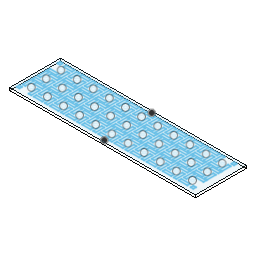
Cable Housing v2 (Autodesk Fusion 360 archive; units mm, degrees)
design "shelf small"
Autodesk Fusion 360 part; units mm, degrees
sketch "Sketch1" plane through (0, 0, 0) normal (0, 0, 1) x (1, 0, 0)
  line L0 (109.5, -30) -> (-109.5, -30)
  line L1 (-109.5, -30) -> (-109.5, 30)
  line L2 (-109.5, 30) -> (109.5, 30)
  line L3 (109.5, 30) -> (109.5, -30)
  line L4 (109.5, -30) -> (-109.5, 30) construction
  line L5 (-109.5, -30) -> (109.5, 30) construction
  dimension "d1" = 60
  dimension "d2" = 219
  constraint horizontal L0
  constraint perpendicular L0 L1
  constraint parallel L0 L2
  constraint parallel L1 L3
  constraint coincident L4 origin
  constraint coincident L5 origin
  measures "d1" distance of L0.end L1.end
  measures "d2" distance of L1.end L2.end
extrude "Extrude1" add sketch "Sketch1" along normal blind 3
sketch "Sketch5" plane through (0, 0, 3) normal (0, 0, 1) x (-1, 0, 0)
  line L0 (-109.5, -30) -> (109.5, -30)
  line L1 (109.5, -30) -> (109.5, 30)
  line L2 (109.5, 30) -> (-109.5, 30)
  line L3 (-109.5, 30) -> (-109.5, -30)
  circle A0 centre (97, 17) radius 1.5
  line L4 (99, 9) -> (89, 9)
  line L5 (89, 9) -> (89, 12)
  line L6 (89, 12) -> (99, 12)
  line L7 (99, 12) -> (99, 9)
  line L8 (92, 15) -> (89, 15)
  line L9 (89, 15) -> (89, 25)
  line L10 (89, 25) -> (92, 25)
  line L11 (92, 25) -> (92, 15)
  line L12 (102, 19) -> (105, 19)
  line L13 (105, 19) -> (105, 9)
  line L14 (105, 9) -> (102, 9)
  line L15 (102, 9) -> (102, 19)
  line L16 (70, 15) -> (70, 25)
  line L17 (73, 25) -> (73, 15)
  line L18 (73, 15) -> (70, 15)
  line L19 (70, 9) -> (70, 12)
  line L20 (86, 9) -> (83, 9)
  line L21 (83, 9) -> (83, 19)
  line L22 (86, 19) -> (86, 9)
  line L23 (83, 19) -> (86, 19)
  line L24 (76, 25) -> (76, 22)
  line L25 (86, 25) -> (76, 25)
  line L26 (86, 22) -> (86, 25)
  line L27 (70, 12) -> (80, 12)
  line L28 (80, 9) -> (70, 9)
  line L29 (80, 12) -> (80, 9)
  circle A1 centre (78, 17) radius 1.5
  line L30 (76, 22) -> (86, 22)
  line L31 (70, 25) -> (73, 25)
  line L32 (51, 15) -> (51, 25)
  line L33 (54, 25) -> (54, 15)
  line L34 (54, 15) -> (51, 15)
  line L35 (51, 9) -> (51, 12)
  line L36 (67, 9) -> (64, 9)
  line L37 (64, 9) -> (64, 19)
  line L38 (67, 19) -> (67, 9)
  line L39 (64, 19) -> (67, 19)
  line L40 (57, 25) -> (57, 22)
  line L41 (67, 25) -> (57, 25)
  line L42 (67, 22) -> (67, 25)
  line L43 (51, 12) -> (61, 12)
  line L44 (61, 9) -> (51, 9)
  line L45 (61, 12) -> (61, 9)
  circle A2 centre (59, 17) radius 1.5
  line L46 (57, 22) -> (67, 22)
  line L47 (51, 25) -> (54, 25)
  line L48 (32, 15) -> (32, 25)
  line L49 (35, 25) -> (35, 15)
  line L50 (35, 15) -> (32, 15)
  line L51 (32, 9) -> (32, 12)
  line L52 (48, 9) -> (45, 9)
  line L53 (45, 9) -> (45, 19)
  line L54 (48, 19) -> (48, 9)
  line L55 (45, 19) -> (48, 19)
  line L56 (38, 25) -> (38, 22)
  line L57 (48, 25) -> (38, 25)
  line L58 (48, 22) -> (48, 25)
  line L59 (32, 12) -> (42, 12)
  line L60 (42, 9) -> (32, 9)
  line L61 (42, 12) -> (42, 9)
  circle A3 centre (40, 17) radius 1.5
  line L62 (38, 22) -> (48, 22)
  line L63 (32, 25) -> (35, 25)
  line L64 (13, 15) -> (13, 25)
  line L65 (16, 25) -> (16, 15)
  line L66 (16, 15) -> (13, 15)
  line L67 (13, 9) -> (13, 12)
  line L68 (29, 9) -> (26, 9)
  line L69 (26, 9) -> (26, 19)
  line L70 (29, 19) -> (29, 9)
  line L71 (26, 19) -> (29, 19)
  line L72 (19, 25) -> (19, 22)
  line L73 (29, 25) -> (19, 25)
  line L74 (29, 22) -> (29, 25)
  line L75 (13, 12) -> (23, 12)
  line L76 (23, 9) -> (13, 9)
  line L77 (23, 12) -> (23, 9)
  circle A4 centre (21, 17) radius 1.5
  line L78 (19, 22) -> (29, 22)
  line L79 (13, 25) -> (16, 25)
  line L80 (-6, 15) -> (-6, 25)
  line L81 (-3, 25) -> (-3, 15)
  line L82 (-3, 15) -> (-6, 15)
  line L83 (-6, 9) -> (-6, 12)
  line L84 (10, 9) -> (7, 9)
  line L85 (7, 9) -> (7, 19)
  line L86 (10, 19) -> (10, 9)
  line L87 (7, 19) -> (10, 19)
  line L88 (0, 25) -> (0, 22)
  line L89 (10, 25) -> (0, 25)
  line L90 (10, 22) -> (10, 25)
  line L91 (-6, 12) -> (4, 12)
  line L92 (4, 9) -> (-6, 9)
  line L93 (4, 12) -> (4, 9)
  circle A5 centre (2, 17) radius 1.5
  line L94 (0, 22) -> (10, 22)
  line L95 (-6, 25) -> (-3, 25)
  line L96 (-25, 15) -> (-25, 25)
  line L97 (-22, 25) -> (-22, 15)
  line L98 (-22, 15) -> (-25, 15)
  line L99 (-25, 9) -> (-25, 12)
  line L100 (-9, 9) -> (-12, 9)
  line L101 (-12, 9) -> (-12, 19)
  line L102 (-9, 19) -> (-9, 9)
  line L103 (-12, 19) -> (-9, 19)
  line L104 (-19, 25) -> (-19, 22)
  line L105 (-9, 25) -> (-19, 25)
  line L106 (-9, 22) -> (-9, 25)
  line L107 (-25, 12) -> (-15, 12)
  line L108 (-15, 9) -> (-25, 9)
  line L109 (-15, 12) -> (-15, 9)
  circle A6 centre (-17, 17) radius 1.5
  line L110 (-19, 22) -> (-9, 22)
  line L111 (-25, 25) -> (-22, 25)
  line L112 (-44, 15) -> (-44, 25)
  line L113 (-41, 25) -> (-41, 15)
  line L114 (-41, 15) -> (-44, 15)
  line L115 (-44, 9) -> (-44, 12)
  line L116 (-28, 9) -> (-31, 9)
  line L117 (-31, 9) -> (-31, 19)
  line L118 (-28, 19) -> (-28, 9)
  line L119 (-31, 19) -> (-28, 19)
  line L120 (-38, 25) -> (-38, 22)
  line L121 (-28, 25) -> (-38, 25)
  line L122 (-28, 22) -> (-28, 25)
  line L123 (-44, 12) -> (-34, 12)
  line L124 (-34, 9) -> (-44, 9)
  line L125 (-34, 12) -> (-34, 9)
  circle A7 centre (-36, 17) radius 1.5
  line L126 (-38, 22) -> (-28, 22)
  line L127 (-44, 25) -> (-41, 25)
  line L128 (-63, 15) -> (-63, 25)
  line L129 (-60, 25) -> (-60, 15)
  line L130 (-60, 15) -> (-63, 15)
  line L131 (-63, 9) -> (-63, 12)
  line L132 (-47, 9) -> (-50, 9)
  line L133 (-50, 9) -> (-50, 19)
  line L134 (-47, 19) -> (-47, 9)
  line L135 (-50, 19) -> (-47, 19)
  line L136 (-57, 25) -> (-57, 22)
  line L137 (-47, 25) -> (-57, 25)
  line L138 (-47, 22) -> (-47, 25)
  line L139 (-63, 12) -> (-53, 12)
  line L140 (-53, 9) -> (-63, 9)
  line L141 (-53, 12) -> (-53, 9)
  circle A8 centre (-55, 17) radius 1.5
  line L142 (-57, 22) -> (-47, 22)
  line L143 (-63, 25) -> (-60, 25)
  line L144 (-82, 15) -> (-82, 25)
  line L145 (-79, 25) -> (-79, 15)
  line L146 (-79, 15) -> (-82, 15)
  line L147 (-82, 9) -> (-82, 12)
  line L148 (-66, 9) -> (-69, 9)
  line L149 (-69, 9) -> (-69, 19)
  line L150 (-66, 19) -> (-66, 9)
  line L151 (-69, 19) -> (-66, 19)
  line L152 (-76, 25) -> (-76, 22)
  line L153 (-66, 25) -> (-76, 25)
  line L154 (-66, 22) -> (-66, 25)
  line L155 (-82, 12) -> (-72, 12)
  line L156 (-72, 9) -> (-82, 9)
  line L157 (-72, 12) -> (-72, 9)
  circle A9 centre (-74, 17) radius 1.5
  line L158 (-76, 22) -> (-66, 22)
  line L159 (-82, 25) -> (-79, 25)
  line L160 (-101, 9) -> (-101, 12)
  line L161 (-85, 9) -> (-88, 9)
  line L162 (-88, 9) -> (-88, 19)
  line L163 (-85, 19) -> (-85, 9)
  line L164 (-88, 19) -> (-85, 19)
  line L165 (-95, 25) -> (-95, 22)
  line L166 (-85, 25) -> (-95, 25)
  line L167 (-85, 22) -> (-85, 25)
  line L168 (-101, 12) -> (-91, 12)
  line L169 (-91, 9) -> (-101, 9)
  line L170 (-91, 12) -> (-91, 9)
  circle A10 centre (-93, 17) radius 1.5
  line L171 (-95, 22) -> (-85, 22)
  line L172 (89, -2.5) -> (89, 7.5)
  line L173 (92, 7.5) -> (92, -2.5)
  line L174 (92, -2.5) -> (89, -2.5)
  line L175 (89, -8.5) -> (89, -5.5)
  line L176 (105, -8.5) -> (102, -8.5)
  line L177 (102, -8.5) -> (102, 1.5)
  line L178 (105, 1.5) -> (105, -8.5)
  line L179 (102, 1.5) -> (105, 1.5)
  line L180 (95, 7.5) -> (95, 4.5)
  line L181 (105, 7.5) -> (95, 7.5)
  line L182 (105, 4.5) -> (105, 7.5)
  line L183 (89, -5.5) -> (99, -5.5)
  line L184 (99, -8.5) -> (89, -8.5)
  line L185 (99, -5.5) -> (99, -8.5)
  circle A11 centre (97, -0.5) radius 1.5
  line L186 (95, 4.5) -> (105, 4.5)
  line L187 (89, 7.5) -> (92, 7.5)
  line L188 (70, -2.5) -> (70, 7.5)
  line L189 (73, 7.5) -> (73, -2.5)
  line L190 (73, -2.5) -> (70, -2.5)
  line L191 (70, -8.5) -> (70, -5.5)
  line L192 (86, -8.5) -> (83, -8.5)
  line L193 (83, -8.5) -> (83, 1.5)
  line L194 (86, 1.5) -> (86, -8.5)
  line L195 (83, 1.5) -> (86, 1.5)
  line L196 (76, 7.5) -> (76, 4.5)
  line L197 (86, 7.5) -> (76, 7.5)
  line L198 (86, 4.5) -> (86, 7.5)
  line L199 (70, -5.5) -> (80, -5.5)
  line L200 (80, -8.5) -> (70, -8.5)
  line L201 (80, -5.5) -> (80, -8.5)
  circle A12 centre (78, -0.5) radius 1.5
  line L202 (76, 4.5) -> (86, 4.5)
  line L203 (70, 7.5) -> (73, 7.5)
  line L204 (51, -2.5) -> (51, 7.5)
  line L205 (54, 7.5) -> (54, -2.5)
  line L206 (54, -2.5) -> (51, -2.5)
  line L207 (51, -8.5) -> (51, -5.5)
  line L208 (67, -8.5) -> (64, -8.5)
  line L209 (64, -8.5) -> (64, 1.5)
  line L210 (67, 1.5) -> (67, -8.5)
  line L211 (64, 1.5) -> (67, 1.5)
  line L212 (57, 7.5) -> (57, 4.5)
  line L213 (67, 7.5) -> (57, 7.5)
  line L214 (67, 4.5) -> (67, 7.5)
  line L215 (51, -5.5) -> (61, -5.5)
  line L216 (61, -8.5) -> (51, -8.5)
  line L217 (61, -5.5) -> (61, -8.5)
  circle A13 centre (59, -0.5) radius 1.5
  line L218 (57, 4.5) -> (67, 4.5)
  line L219 (51, 7.5) -> (54, 7.5)
  line L220 (32, -2.5) -> (32, 7.5)
  line L221 (35, 7.5) -> (35, -2.5)
  line L222 (35, -2.5) -> (32, -2.5)
  line L223 (32, -8.5) -> (32, -5.5)
  line L224 (48, -8.5) -> (45, -8.5)
  line L225 (45, -8.5) -> (45, 1.5)
  line L226 (48, 1.5) -> (48, -8.5)
  line L227 (45, 1.5) -> (48, 1.5)
  line L228 (38, 7.5) -> (38, 4.5)
  line L229 (48, 7.5) -> (38, 7.5)
  line L230 (48, 4.5) -> (48, 7.5)
  line L231 (32, -5.5) -> (42, -5.5)
  line L232 (42, -8.5) -> (32, -8.5)
  line L233 (42, -5.5) -> (42, -8.5)
  circle A14 centre (40, -0.5) radius 1.5
  line L234 (38, 4.5) -> (48, 4.5)
  line L235 (32, 7.5) -> (35, 7.5)
  line L236 (13, -2.5) -> (13, 7.5)
  line L237 (16, 7.5) -> (16, -2.5)
  line L238 (16, -2.5) -> (13, -2.5)
  line L239 (13, -8.5) -> (13, -5.5)
  line L240 (29, -8.5) -> (26, -8.5)
  line L241 (26, -8.5) -> (26, 1.5)
  line L242 (29, 1.5) -> (29, -8.5)
  line L243 (26, 1.5) -> (29, 1.5)
  line L244 (19, 7.5) -> (19, 4.5)
  line L245 (29, 7.5) -> (19, 7.5)
  line L246 (29, 4.5) -> (29, 7.5)
  line L247 (13, -5.5) -> (23, -5.5)
  line L248 (23, -8.5) -> (13, -8.5)
  line L249 (23, -5.5) -> (23, -8.5)
  circle A15 centre (21, -0.5) radius 1.5
  line L250 (19, 4.5) -> (29, 4.5)
  line L251 (13, 7.5) -> (16, 7.5)
  line L252 (-6, -2.5) -> (-6, 7.5)
  line L253 (-3, 7.5) -> (-3, -2.5)
  line L254 (-3, -2.5) -> (-6, -2.5)
  line L255 (-6, -8.5) -> (-6, -5.5)
  line L256 (10, -8.5) -> (7, -8.5)
  line L257 (7, -8.5) -> (7, 1.5)
  line L258 (10, 1.5) -> (10, -8.5)
  line L259 (7, 1.5) -> (10, 1.5)
  line L260 (0, 7.5) -> (0, 4.5)
  line L261 (10, 7.5) -> (0, 7.5)
  line L262 (10, 4.5) -> (10, 7.5)
  line L263 (-6, -5.5) -> (4, -5.5)
  line L264 (4, -8.5) -> (-6, -8.5)
  line L265 (4, -5.5) -> (4, -8.5)
  circle A16 centre (2, -0.5) radius 1.5
  line L266 (0, 4.5) -> (10, 4.5)
  line L267 (-6, 7.5) -> (-3, 7.5)
  line L268 (-25, -2.5) -> (-25, 7.5)
  line L269 (-22, 7.5) -> (-22, -2.5)
  line L270 (-22, -2.5) -> (-25, -2.5)
  line L271 (-25, -8.5) -> (-25, -5.5)
  line L272 (-9, -8.5) -> (-12, -8.5)
  line L273 (-12, -8.5) -> (-12, 1.5)
  line L274 (-9, 1.5) -> (-9, -8.5)
  line L275 (-12, 1.5) -> (-9, 1.5)
  line L276 (-19, 7.5) -> (-19, 4.5)
  line L277 (-9, 7.5) -> (-19, 7.5)
  line L278 (-9, 4.5) -> (-9, 7.5)
  line L279 (-25, -5.5) -> (-15, -5.5)
  line L280 (-15, -8.5) -> (-25, -8.5)
  line L281 (-15, -5.5) -> (-15, -8.5)
  circle A17 centre (-17, -0.5) radius 1.5
  line L282 (-19, 4.5) -> (-9, 4.5)
  line L283 (-25, 7.5) -> (-22, 7.5)
  line L284 (-44, -2.5) -> (-44, 7.5)
  line L285 (-41, 7.5) -> (-41, -2.5)
  line L286 (-41, -2.5) -> (-44, -2.5)
  line L287 (-44, -8.5) -> (-44, -5.5)
  line L288 (-28, -8.5) -> (-31, -8.5)
  line L289 (-31, -8.5) -> (-31, 1.5)
  line L290 (-28, 1.5) -> (-28, -8.5)
  line L291 (-31, 1.5) -> (-28, 1.5)
  line L292 (-38, 7.5) -> (-38, 4.5)
  line L293 (-28, 7.5) -> (-38, 7.5)
  line L294 (-28, 4.5) -> (-28, 7.5)
  line L295 (-44, -5.5) -> (-34, -5.5)
  line L296 (-34, -8.5) -> (-44, -8.5)
  line L297 (-34, -5.5) -> (-34, -8.5)
  circle A18 centre (-36, -0.5) radius 1.5
  line L298 (-38, 4.5) -> (-28, 4.5)
  line L299 (-44, 7.5) -> (-41, 7.5)
  line L300 (-63, -2.5) -> (-63, 7.5)
  line L301 (-60, 7.5) -> (-60, -2.5)
  line L302 (-60, -2.5) -> (-63, -2.5)
  line L303 (-63, -8.5) -> (-63, -5.5)
  line L304 (-47, -8.5) -> (-50, -8.5)
  line L305 (-50, -8.5) -> (-50, 1.5)
  line L306 (-47, 1.5) -> (-47, -8.5)
  line L307 (-50, 1.5) -> (-47, 1.5)
  line L308 (-57, 7.5) -> (-57, 4.5)
  line L309 (-47, 7.5) -> (-57, 7.5)
  line L310 (-47, 4.5) -> (-47, 7.5)
  line L311 (-63, -5.5) -> (-53, -5.5)
  line L312 (-53, -8.5) -> (-63, -8.5)
  line L313 (-53, -5.5) -> (-53, -8.5)
  circle A19 centre (-55, -0.5) radius 1.5
  line L314 (-57, 4.5) -> (-47, 4.5)
  line L315 (-63, 7.5) -> (-60, 7.5)
  line L316 (-82, -2.5) -> (-82, 7.5)
  line L317 (-79, 7.5) -> (-79, -2.5)
  line L318 (-79, -2.5) -> (-82, -2.5)
  line L319 (-82, -8.5) -> (-82, -5.5)
  line L320 (-66, -8.5) -> (-69, -8.5)
  line L321 (-69, -8.5) -> (-69, 1.5)
  line L322 (-66, 1.5) -> (-66, -8.5)
  line L323 (-69, 1.5) -> (-66, 1.5)
  line L324 (-76, 7.5) -> (-76, 4.5)
  line L325 (-66, 7.5) -> (-76, 7.5)
  line L326 (-66, 4.5) -> (-66, 7.5)
  line L327 (-82, -5.5) -> (-72, -5.5)
  line L328 (-72, -8.5) -> (-82, -8.5)
  line L329 (-72, -5.5) -> (-72, -8.5)
  circle A20 centre (-74, -0.5) radius 1.5
  line L330 (-76, 4.5) -> (-66, 4.5)
  line L331 (-82, 7.5) -> (-79, 7.5)
  line L332 (-101, -2.5) -> (-101, 7.5)
  line L333 (-98, 7.5) -> (-98, -2.5)
  line L334 (-98, -2.5) -> (-101, -2.5)
  line L335 (-101, -8.5) -> (-101, -5.5)
  line L336 (-85, -8.5) -> (-88, -8.5)
  line L337 (-88, -8.5) -> (-88, 1.5)
  line L338 (-85, 1.5) -> (-85, -8.5)
  line L339 (-88, 1.5) -> (-85, 1.5)
  line L340 (-95, 7.5) -> (-95, 4.5)
  line L341 (-85, 7.5) -> (-95, 7.5)
  line L342 (-85, 4.5) -> (-85, 7.5)
  line L343 (-101, -5.5) -> (-91, -5.5)
  line L344 (-91, -8.5) -> (-101, -8.5)
  line L345 (-91, -5.5) -> (-91, -8.5)
  circle A21 centre (-93, -0.5) radius 1.5
  line L346 (-95, 4.5) -> (-85, 4.5)
  line L347 (-101, 7.5) -> (-98, 7.5)
  line L348 (89, -20) -> (89, -10)
  line L349 (92, -10) -> (92, -20)
  line L350 (92, -20) -> (89, -20)
  line L351 (89, -26) -> (89, -23)
  line L352 (95, -10) -> (95, -13)
  line L353 (105, -10) -> (95, -10)
  line L354 (105, -13) -> (105, -10)
  line L355 (89, -23) -> (99, -23)
  line L356 (99, -26) -> (89, -26)
  line L357 (99, -23) -> (99, -26)
  circle A22 centre (97, -18) radius 1.5
  line L358 (95, -13) -> (105, -13)
  line L359 (89, -10) -> (92, -10)
  line L360 (70, -20) -> (70, -10)
  line L361 (73, -10) -> (73, -20)
  line L362 (73, -20) -> (70, -20)
  line L363 (70, -26) -> (70, -23)
  line L364 (86, -26) -> (83, -26)
  line L365 (83, -26) -> (83, -16)
  line L366 (86, -16) -> (86, -26)
  line L367 (83, -16) -> (86, -16)
  line L368 (76, -10) -> (76, -13)
  line L369 (86, -10) -> (76, -10)
  line L370 (86, -13) -> (86, -10)
  line L371 (70, -23) -> (80, -23)
  line L372 (80, -26) -> (70, -26)
  line L373 (80, -23) -> (80, -26)
  circle A23 centre (78, -18) radius 1.5
  line L374 (76, -13) -> (86, -13)
  line L375 (70, -10) -> (73, -10)
  line L376 (51, -20) -> (51, -10)
  line L377 (54, -10) -> (54, -20)
  line L378 (54, -20) -> (51, -20)
  line L379 (51, -26) -> (51, -23)
  line L380 (67, -26) -> (64, -26)
  line L381 (64, -26) -> (64, -16)
  line L382 (67, -16) -> (67, -26)
  line L383 (64, -16) -> (67, -16)
  line L384 (57, -10) -> (57, -13)
  line L385 (67, -10) -> (57, -10)
  line L386 (67, -13) -> (67, -10)
  line L387 (51, -23) -> (61, -23)
  line L388 (61, -26) -> (51, -26)
  line L389 (61, -23) -> (61, -26)
  circle A24 centre (59, -18) radius 1.5
  line L390 (57, -13) -> (67, -13)
  line L391 (51, -10) -> (54, -10)
  line L392 (32, -20) -> (32, -10)
  line L393 (35, -10) -> (35, -20)
  line L394 (35, -20) -> (32, -20)
  line L395 (32, -26) -> (32, -23)
  line L396 (48, -26) -> (45, -26)
  line L397 (45, -26) -> (45, -16)
  line L398 (48, -16) -> (48, -26)
  line L399 (45, -16) -> (48, -16)
  line L400 (38, -10) -> (38, -13)
  line L401 (48, -10) -> (38, -10)
  line L402 (48, -13) -> (48, -10)
  line L403 (32, -23) -> (42, -23)
  line L404 (42, -26) -> (32, -26)
  line L405 (42, -23) -> (42, -26)
  circle A25 centre (40, -18) radius 1.5
  line L406 (38, -13) -> (48, -13)
  line L407 (32, -10) -> (35, -10)
  line L408 (13, -20) -> (13, -10)
  line L409 (16, -10) -> (16, -20)
  line L410 (16, -20) -> (13, -20)
  line L411 (13, -26) -> (13, -23)
  line L412 (29, -26) -> (26, -26)
  line L413 (26, -26) -> (26, -16)
  line L414 (29, -16) -> (29, -26)
  line L415 (26, -16) -> (29, -16)
  line L416 (19, -10) -> (19, -13)
  line L417 (29, -10) -> (19, -10)
  line L418 (29, -13) -> (29, -10)
  line L419 (13, -23) -> (23, -23)
  line L420 (23, -26) -> (13, -26)
  line L421 (23, -23) -> (23, -26)
  circle A26 centre (21, -18) radius 1.5
  line L422 (19, -13) -> (29, -13)
  line L423 (13, -10) -> (16, -10)
  line L424 (-6, -20) -> (-6, -10)
  line L425 (-3, -10) -> (-3, -20)
  line L426 (-3, -20) -> (-6, -20)
  line L427 (-6, -26) -> (-6, -23)
  line L428 (10, -26) -> (7, -26)
  line L429 (7, -26) -> (7, -16)
  line L430 (10, -16) -> (10, -26)
  line L431 (7, -16) -> (10, -16)
  line L432 (0, -10) -> (0, -13)
  line L433 (10, -10) -> (0, -10)
  line L434 (10, -13) -> (10, -10)
  line L435 (-6, -23) -> (4, -23)
  line L436 (4, -26) -> (-6, -26)
  line L437 (4, -23) -> (4, -26)
  circle A27 centre (2, -18) radius 1.5
  line L438 (0, -13) -> (10, -13)
  line L439 (-6, -10) -> (-3, -10)
  line L440 (-25, -20) -> (-25, -10)
  line L441 (-22, -10) -> (-22, -20)
  line L442 (-22, -20) -> (-25, -20)
  line L443 (-25, -26) -> (-25, -23)
  line L444 (-9, -26) -> (-12, -26)
  line L445 (-12, -26) -> (-12, -16)
  line L446 (-9, -16) -> (-9, -26)
  line L447 (-12, -16) -> (-9, -16)
  line L448 (-19, -10) -> (-19, -13)
  line L449 (-9, -10) -> (-19, -10)
  line L450 (-9, -13) -> (-9, -10)
  line L451 (-25, -23) -> (-15, -23)
  line L452 (-15, -26) -> (-25, -26)
  line L453 (-15, -23) -> (-15, -26)
  circle A28 centre (-17, -18) radius 1.5
  line L454 (-19, -13) -> (-9, -13)
  line L455 (-25, -10) -> (-22, -10)
  line L456 (-44, -20) -> (-44, -10)
  line L457 (-41, -10) -> (-41, -20)
  line L458 (-41, -20) -> (-44, -20)
  line L459 (-44, -26) -> (-44, -23)
  line L460 (-28, -26) -> (-31, -26)
  line L461 (-31, -26) -> (-31, -16)
  line L462 (-28, -16) -> (-28, -26)
  line L463 (-31, -16) -> (-28, -16)
  line L464 (-38, -10) -> (-38, -13)
  line L465 (-28, -10) -> (-38, -10)
  line L466 (-28, -13) -> (-28, -10)
  line L467 (-44, -23) -> (-34, -23)
  line L468 (-34, -26) -> (-44, -26)
  line L469 (-34, -23) -> (-34, -26)
  circle A29 centre (-36, -18) radius 1.5
  line L470 (-38, -13) -> (-28, -13)
  line L471 (-44, -10) -> (-41, -10)
  line L472 (-63, -20) -> (-63, -10)
  line L473 (-60, -10) -> (-60, -20)
  line L474 (-60, -20) -> (-63, -20)
  line L475 (-63, -26) -> (-63, -23)
  line L476 (-47, -26) -> (-50, -26)
  line L477 (-50, -26) -> (-50, -16)
  line L478 (-47, -16) -> (-47, -26)
  line L479 (-50, -16) -> (-47, -16)
  line L480 (-57, -10) -> (-57, -13)
  line L481 (-47, -10) -> (-57, -10)
  line L482 (-47, -13) -> (-47, -10)
  line L483 (-63, -23) -> (-53, -23)
  line L484 (-53, -26) -> (-63, -26)
  line L485 (-53, -23) -> (-53, -26)
  circle A30 centre (-55, -18) radius 1.5
  line L486 (-57, -13) -> (-47, -13)
  line L487 (-63, -10) -> (-60, -10)
  line L488 (-82, -20) -> (-82, -10)
  line L489 (-79, -10) -> (-79, -20)
  line L490 (-79, -20) -> (-82, -20)
  line L491 (-82, -26) -> (-82, -23)
  line L492 (-66, -26) -> (-69, -26)
  line L493 (-69, -26) -> (-69, -16)
  line L494 (-66, -16) -> (-66, -26)
  line L495 (-69, -16) -> (-66, -16)
  line L496 (-76, -10) -> (-76, -13)
  line L497 (-66, -10) -> (-76, -10)
  line L498 (-66, -13) -> (-66, -10)
  line L499 (-82, -23) -> (-72, -23)
  line L500 (-72, -26) -> (-82, -26)
  line L501 (-72, -23) -> (-72, -26)
  circle A31 centre (-74, -18) radius 1.5
  line L502 (-76, -13) -> (-66, -13)
  line L503 (-82, -10) -> (-79, -10)
  line L504 (-101, -20) -> (-101, -10)
  line L505 (-98, -10) -> (-98, -20)
  line L506 (-98, -20) -> (-101, -20)
  line L507 (-85, -26) -> (-88, -26)
  line L508 (-88, -26) -> (-88, -16)
  line L509 (-85, -16) -> (-85, -26)
  line L510 (-88, -16) -> (-85, -16)
  line L511 (-95, -10) -> (-95, -13)
  line L512 (-85, -10) -> (-95, -10)
  line L513 (-85, -13) -> (-85, -10)
  circle A32 centre (-93, -18) radius 1.5
  line L514 (-95, -13) -> (-85, -13)
  line L515 (-101, -10) -> (-98, -10)
  dimension "d128" = 3
  dimension "d129" = 10
  dimension "d130" = 3
  dimension "d132" = 3
  dimension "d133" = 10
  dimension "d137" = 3
  dimension "d138" = 10
  dimension "d141" = 5
  dimension "d142" = 3
  dimension "d145" = 3
  dimension "d146" = 5
  dimension "d148" = 5
  constraint horizontal L4
  constraint vertical L5
  constraint horizontal L6
  constraint vertical L7
  constraint horizontal L8
  constraint vertical L9
  constraint horizontal L10
  constraint vertical L11
  constraint horizontal L12
  constraint vertical L13
  constraint horizontal L14
  constraint vertical L15
  measures "d128" diameter of A0
  measures "d129" distance of L4.start L4.end
  measures "d130" distance of L4.start L6.end
  measures "d132" distance of L8.start L8.end
  measures "d133" distance of L8.start L10.end
  measures "d137" distance of L12.start L12.end
  measures "d138" distance of L12.start L14.end
  measures "d141" vertical distance of A0.centre L6.end
  measures "d142" vertical distance of L5.end L8.end
  measures "d145" horizontal distance of L4.start L14.end
  measures "d146" distance of A0.centre L11
  measures "d148" distance of A0.centre L15
sketch "Sketch6" plane through (0, 0, 3) normal (0, 0, 1) x (-1, 0, 0)
  line L0 (103, -23) -> (106, -23)
  line L1 (106, -23) -> (106, -26)
  line L2 (106, -26) -> (103, -26)
  line L3 (103, -26) -> (103, -23)
  line L4 (103, 25) -> (106, 25)
  line L5 (106, 25) -> (106, 22)
  line L6 (106, 22) -> (103, 22)
  line L7 (103, 22) -> (103, 25)
  line L8 (-102, 25) -> (-99, 25)
  line L9 (-99, 25) -> (-99, 22)
  line L10 (-99, 22) -> (-102, 22)
  line L11 (-102, 22) -> (-102, 25)
  line L12 (-99, -26) -> (-102, -26)
  line L13 (-102, -26) -> (-102, -23)
  line L14 (-102, -23) -> (-99, -23)
  line L15 (-99, -23) -> (-99, -26)
  line L16 (-1.5, -26.5) -> (1.5, -26.5)
  line L17 (1.5, -26.5) -> (1.5, -29.5)
  line L18 (1.5, -29.5) -> (-1.5, -29.5)
  line L19 (-1.5, -29.5) -> (-1.5, -26.5)
  line L20 (-1.5, -26.5) -> (1.5, -29.5) construction
  line L21 (1.5, -26.5) -> (-1.5, -29.5) construction
  line L22 (-1.5, 29.5) -> (1.5, 29.5)
  line L23 (1.5, 29.5) -> (1.5, 26.5)
  line L24 (1.5, 26.5) -> (-1.5, 26.5)
  line L25 (-1.5, 26.5) -> (-1.5, 29.5)
  line L26 (-1.5, 29.5) -> (1.5, 26.5) construction
  line L27 (1.5, 29.5) -> (-1.5, 26.5) construction
  point P0 (0, -28)
  point P1 (0, 28)
  dimension "d153" = 3
  dimension "d154" = 3
  dimension "d155" = 3
  dimension "d156" = 3
  constraint horizontal L0
  constraint vertical L1
  constraint horizontal L2
  constraint vertical L3
  constraint horizontal L4
  constraint vertical L5
  constraint horizontal L6
  constraint vertical L7
  constraint horizontal L8
  constraint vertical L9
  constraint horizontal L10
  constraint vertical L11
  constraint horizontal L12
  constraint vertical L13
  constraint horizontal L14
  constraint vertical L15
  constraint horizontal L16
  constraint perpendicular L16 L17
  constraint parallel L16 L18
  constraint parallel L17 L19
  constraint coincident L20 P0
  constraint coincident L21 P0
  constraint horizontal L22
  constraint perpendicular L22 L23
  constraint parallel L22 L24
  constraint parallel L23 L25
  constraint coincident L26 P1
  constraint coincident L27 P1
  measures "d153" distance of L17.end L18.end
  measures "d154" distance of L16.end L17.end
  measures "d155" distance of L23.end L24.end
  measures "d156" distance of L22.end L23.end
extrude "Extrude2" [rolled back] along distance -5 taper angle 0
extrude "Extrude3" [rolled back] along distance -5 taper angle 0
